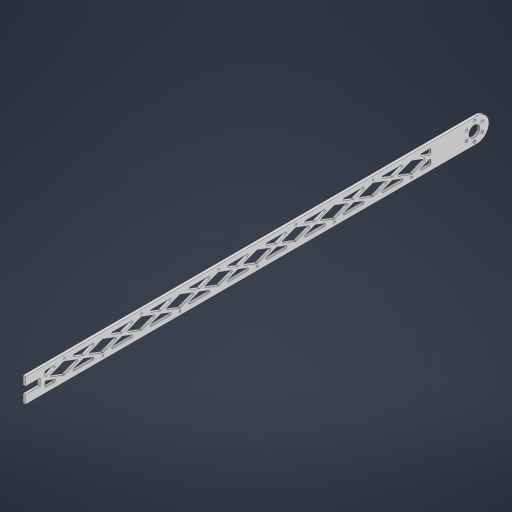
# Autodesk Inventor part: Arm
Saved by Autodesk Inventor 2023 (Build 270158000, 158)
## iProperties
Created: 2023-01-21
Part Number: Arm
Material: Generic
Document SubType Name: Modeling
Designer: Terrence
Density: 1 g/cm^3
Appearance: Default
Author: Terrence
Autodesk Inventor part; units mm, degrees
ref_plane "YZ Plane" through (0, 0, 0) normal (1, 0, 0) x (0, 1, 0)
ref_plane "XZ Plane" through (0, 0, 0) normal (0, 1, 0) x (-1, 0, 0)
ref_plane "XY Plane" through (0, 0, 0) normal (0, 0, 1) x (1, 0, 0)
sketch "Sketch1" plane through (0, 0, 0) normal (1, 0, 0) x (0, 1, 0)
  line L0 (0, 25.4) -> (63.5, 25.4)
  line L1 (63.5, 25.4) -> (63.5, -1193.8)
  line L2 (63.5, -1193.8) -> (0, -1193.8)
  line L3 (0, -1193.8) -> (0, 25.4)
  dimension "d0" = 63.5
  dimension "d1" = 1219.2
  constraints: 8 end point, 2 parallel, 1 horizontal, 1 perpendicular, 1 other
  measures "d0" distance of L1.end L2.end
  measures "d1" distance of L0.end L1.end
extrude "Extrusion1" add sketch "Sketch1" along normal blind 6.35
sketch "Sketch2" plane through (6.35, 0, 0) normal (1, 0, 0) x (0, 0, -1)
  line L0 (1193.8, 63.5) -> (-25.4, 63.5) projected
  line L1 (1155.7, 63.5) -> (1155.7, 0) construction
  line L2 (0, 0) -> (1193.8, 0) projected
  circle A0 centre (1155.7, 31.75) radius 14.2875
  dimension "d5" = 1155.7
  dimension "d24" = 28.575
  constraints: 2 end point, 2 point on line, 1 centre point, 1 midpoint, 1 perpendicular
  measures "d5" distance from line of L2.start L1
  measures "d24" diameter of A0
extrude "Extrusion2" cut sketch "Sketch2" against normal through all
fillet "Fillet1" radius 31.75 2 edges at (3.175, 63.5, -1193.8) (3.175, 0, -1193.8)
sketch "Sketch3" plane through (6.35, 0, 0) normal (1, 0, 0) x (0, 0, -1)
  line L0 (25.4, 50.8) -> (1041.4, 50.8)
  line L1 (1041.4, 50.8) -> (1041.4, 12.7)
  line L2 (1041.4, 12.7) -> (25.4, 12.7)
  line L3 (25.4, 12.7) -> (25.4, 50.8)
  line L4 (0, 0) -> (1162.05, 0) projected
  line L5 (1162.05, 63.5) -> (-25.4, 63.5) projected
  line L6 (-25.4, 63.5) -> (-25.4, 0) projected
  dimension "d9" = 12.7
  dimension "d10" = 12.7
  dimension "d11" = 50.8
  dimension "d12" = 1016
  constraints: 8 end point, 2 parallel, 1 horizontal, 1 perpendicular
  measures "d9" distance between parallel lines of L4 L2
  measures "d10" distance between parallel lines of L5 L0
  measures "d11" distance between parallel lines of L6 L3
  measures "d12" distance of L1.end L2.end
extrude "Extrusion3" cut sketch "Sketch3" against normal through all
sketch "Sketch4" plane through (6.35, 0, 0) normal (1, 0, 0) x (0, 0, -1)
  line L0 (25.4, 50.8) -> (127, 50.8) construction
  line L1 (127, 50.8) -> (127, 12.7) construction
  line L2 (127, 12.7) -> (25.4, 12.7) construction
  line L3 (25.4, 12.7) -> (25.4, 50.8) construction
  line L4 (25.4, 31.75) -> (76.2, 50.8) construction
  line L5 (76.2, 50.8) -> (127, 31.75) construction
  line L6 (127, 31.75) -> (76.2, 12.7) construction
  line L7 (76.2, 12.7) -> (25.4, 31.75) construction
  line L8 (24.2852, 34.7228) -> (75.0852, 53.7728)
  line L9 (75.0852, 53.7728) -> (77.3148, 47.8272)
  line L10 (77.3148, 47.8272) -> (26.5148, 28.7772)
  line L11 (26.5148, 28.7772) -> (24.2852, 34.7228)
  line L12 (24.2852, 34.7228) -> (77.3148, 47.8272) construction
  line L13 (75.0852, 53.7728) -> (26.5148, 28.7772) construction
  line L14 (128.1148, 34.7228) -> (77.3148, 53.7728)
  line L15 (77.3148, 53.7728) -> (75.0852, 47.8272)
  line L16 (75.0852, 47.8272) -> (125.8852, 28.7772)
  line L17 (125.8852, 28.7772) -> (128.1148, 34.7228)
  line L18 (128.1148, 34.7228) -> (75.0852, 47.8272) construction
  line L19 (77.3148, 53.7728) -> (125.8852, 28.7772) construction
  line L20 (24.2852, 28.7772) -> (75.0852, 9.7272)
  line L21 (75.0852, 9.7272) -> (77.3148, 15.6728)
  line L22 (77.3148, 15.6728) -> (26.5148, 34.7228)
  line L23 (26.5148, 34.7228) -> (24.2852, 28.7772)
  line L24 (24.2852, 28.7772) -> (77.3148, 15.6728) construction
  line L25 (75.0852, 9.7272) -> (26.5148, 34.7228) construction
  line L26 (75.0852, 15.6728) -> (125.8852, 34.7228)
  line L27 (125.8852, 34.7228) -> (128.1148, 28.7772)
  line L28 (128.1148, 28.7772) -> (77.3148, 9.7272)
  line L29 (77.3148, 9.7272) -> (75.0852, 15.6728)
  line L30 (75.0852, 15.6728) -> (128.1148, 28.7772) construction
  line L31 (125.8852, 34.7228) -> (77.3148, 9.7272) construction
  point P0 (0, 0)
  point P1 (50.8, 41.275)
  point P2 (101.6, 41.275)
  point P3 (50.8, 22.225)
  point P4 (101.6, 22.225)
  point P5 (25.4, 31.75)
  point P6 (76.2, 12.7)
  point P7 (76.2, 47.4091)
  point P8 (117.9576, 31.75)
  point P9 (76.2, 16.0909)
  point P10 (34.4424, 31.75)
  point P11 (76.2, 50.8)
  point P12 (127, 31.75)
  dimension "d15" = 101.6
  dimension "d16" = 6.35
  dimension "d17" = 6.35
  constraints: 64 end point, 22 midpoint, 13 parallel, 5 perpendicular, 2 coincident, 2 equal length, 1 horizontal
  measures "d15" distance of L1.end L2.end
  measures "d16" distance of L8.end L9.end
  measures "d17" distance of L15.end L14.end
extrude "Extrusion4" add sketch "Sketch4" against normal up to surface (6.35 mm away) contours L8 L9 L15 L16 L10 L22 L23 L11 | L23 L22 L10 L11 | L11 L10 L22 L26 L29 L21 L20 L23 | L15 L14 L17 L27 L26 L16 L10 L9 | L9 L10 L16 L15 | L26 L16 L17 L27 L28 L29 L21 L22 | L22 L21 L29 L26 | L26 L27 L17 L16
pattern_linear "Rectangular Pattern1" count 10 spacing 101.6 along (0, 0, -1) of "Extrusion4"
fillet "Fillet2" radius 3.175 106 edges at (3.175, 12.7, -168.7576) (3.175, 12.7, -85.2424) (3.175, 12.7, -270.3576) (3.175, 12.7, -186.8424) (3.175, 12.7, -371.9576) (3.175, 12.7, -288.4424) (3.175, 12.7, -473.5576) (3.175, 12.7, -390.0424) (3.175, 12.7, -575.1576) (3.175, 12.7, -491.6424) (3.175, 12.7, -676.7576) (3.175, 12.7, -593.2424) (3.175, 12.7, -778.3576) (3.175, 12.7, -694.8424) (3.175, 12.7, -879.9576) (3.175, 12.7, -796.4424) (3.175, 12.7, -981.5576) (3.175, 12.7, -898.0424) (3.175, 12.7, -1041.4) (3.175, 12.7, -999.6424) (3.175, 28.3591, -1041.4) (3.175, 50.8, -1041.4) (3.175, 35.1409, -1041.4) (3.175, 50.8, -999.6424) (3.175, 50.8, -898.0424) (3.175, 50.8, -981.5576) (3.175, 50.8, -796.4424) (3.175, 50.8, -879.9576) (3.175, 50.8, -694.8424) (3.175, 50.8, -778.3576) (3.175, 50.8, -593.2424) (3.175, 50.8, -676.7576) (3.175, 50.8, -491.6424) (3.175, 50.8, -575.1576) (3.175, 50.8, -390.0424) (3.175, 50.8, -473.5576) (3.175, 50.8, -288.4424) (3.175, 50.8, -371.9576) (3.175, 50.8, -186.8424) (3.175, 50.8, -270.3576) (3.175, 50.8, -85.2424) (3.175, 50.8, -168.7576) (3.175, 35.1409, -127) (3.175, 28.3591, -127) (3.175, 12.7, -25.4) (3.175, 28.3591, -25.4) (3.175, 12.7, -67.1576) (3.175, 16.0909, -76.2) (3.175, 31.75, -34.4424) (3.175, 31.75, -117.9576) (3.175, 47.4091, -76.2) (3.175, 35.1409, -25.4) (3.175, 50.8, -25.4) (3.175, 50.8, -67.1576) (3.175, 35.1409, -228.6) (3.175, 28.3591, -228.6) (3.175, 47.4091, -177.8) (3.175, 31.75, -219.5576) (3.175, 31.75, -136.0424) (3.175, 16.0909, -177.8) (3.175, 28.3591, -330.2) (3.175, 28.3591, -431.8) (3.175, 28.3591, -533.4) (3.175, 28.3591, -635) (3.175, 28.3591, -736.6) (3.175, 28.3591, -838.2) (3.175, 28.3591, -939.8) (3.175, 35.1409, -939.8) (3.175, 35.1409, -838.2) (3.175, 35.1409, -736.6) (3.175, 35.1409, -635) (3.175, 35.1409, -533.4) (3.175, 35.1409, -431.8) (3.175, 35.1409, -330.2) (3.175, 47.4091, -279.4) (3.175, 31.75, -321.1576) (3.175, 31.75, -237.6424) (3.175, 16.0909, -279.4) (3.175, 47.4091, -381) (3.175, 31.75, -422.7576) (3.175, 31.75, -339.2424) (3.175, 16.0909, -381) (3.175, 47.4091, -482.6) (3.175, 31.75, -524.3576) (3.175, 31.75, -440.8424) (3.175, 16.0909, -482.6) (3.175, 47.4091, -584.2) (3.175, 31.75, -625.9576) (3.175, 31.75, -542.4424) (3.175, 16.0909, -584.2) (3.175, 47.4091, -685.8) (3.175, 31.75, -727.5576) (3.175, 31.75, -644.0424) (3.175, 16.0909, -685.8) (3.175, 47.4091, -787.4) (3.175, 31.75, -829.1576) (3.175, 31.75, -745.6424) (3.175, 16.0909, -787.4) (3.175, 47.4091, -889) (3.175, 31.75, -930.7576) (3.175, 31.75, -847.2424) (3.175, 16.0909, -889) (3.175, 47.4091, -990.6) (3.175, 31.75, -1032.3576) (3.175, 31.75, -948.8424) (3.175, 16.0909, -990.6)
sketch "Sketch5" plane through (6.35, 0, 0) normal (1, 0, 0) x (0, 0, -1)
  circle A0 centre (1155.7, 31.75) radius 14.2875 projected
  line L0 (1155.7, 31.75) -> (1155.7, 55.5752) construction
  circle A1 centre (1155.7, 55.5752) radius 3.6233
  point P0 (0, 0)
  dimension "d32" = 23.8252
  constraints: 2 end point, 1 centre point, 1 coincident, 1 vertical
  measures "d32" distance of L0.start L0.end
extrude "Extrusion5" cut sketch "Sketch5" against normal through all contours A1
pattern_circular "Circular Pattern1" count 6 over 360 about axis through (6.35, 31.75, -1155.7) along (-1, 0, 0) of "Extrusion5"
sketch "Sketch6" plane through (6.35, 0, 0) normal (1, 0, 0) x (0, 0, -1)
  circle A0 centre (76.2, 53.975) radius 2.54
  arc A1 (77.3148, 46.991) -> (75.0852, 46.991) centre (76.2, 44.0182) ccw projected
  line L0 (76.2, 47.1932) -> (76.2, 63.5) construction
  line L1 (1162.05, 63.5) -> (-25.4, 63.5) projected
  line L2 (76.2, 44.0182) -> (76.2, 46.2921) construction
  circle A2 centre (177.8, 9.525) radius 2.54
  arc A3 (176.3801, 16.9597) -> (179.2199, 16.9597) centre (177.8, 19.7995) ccw projected
  line L3 (177.8, 19.7995) -> (177.8, 16.6245)
  line L4 (0, 0) -> (1162.05, 0) projected
  dimension "d33" = 9.525
  dimension "d34" = 5.08
  dimension "d35" = 9.525
  dimension "d36" = 5.08
  constraints: 6 end point, 3 point on line, 3 vertical, 2 centre point, 2 point on circle, 1 collinear
  measures "d33" distance of L0.end A0.centre
  measures "d34" diameter of A0
  measures "d35" distance from line of L4 A2.centre
  measures "d36" diameter of A2
extrude "Extrusion6" cut sketch "Sketch6" against normal through all
pattern_linear "Rectangular Pattern2" count 5 spacing -203.2 along (0, 0, 1) of "Extrusion6"
sketch "Sketch8" plane through (6.35, 0, 0) normal (1, 0, 0) x (0, 0, -1)
  line L0 (-25.4, 41.275) -> (12.7, 41.275)
  line L1 (12.7, 41.275) -> (12.7, 22.225)
  line L2 (12.7, 22.225) -> (-25.4, 22.225)
  line L3 (-25.4, 22.225) -> (-25.4, 41.275)
  line L4 (-25.4, 63.5) -> (-25.4, 0) projected
  point P0 (0, 0)
  point P1 (-25.4, 31.75)
  dimension "d44" = 38.1
  dimension "d45" = 19.05
  constraints: 8 end point, 2 midpoint, 2 parallel, 1 horizontal, 1 perpendicular
  measures "d44" distance of L1.end L2.end
  measures "d45" distance of L2.end L0.start
extrude "Extrusion8" cut sketch "Sketch8" against normal blind 25.4
body "Solid1"
